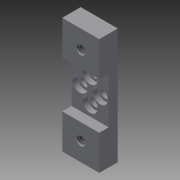
# Autodesk Inventor part: 2750-1_b
Saved by Autodesk Inventor 2014 SP2 (Build 180246200, 246)
## iProperties
Created: 2019-11-08
Part Number: 2750-1_b
Material: Generic
Catalog Web Link: www.cadenas.de
Description: 2750, 2752, 2754, 2757, 2750-Black, 2752-Black, 2754-Black, 2757-Black_b-Roller Wheel Brackets
Vendor: 8020
Document SubType Name: Modeling
Designer: psadmin
Manufacturer: 8020
Mass: 18.3475 g
Surface Area: 73.1333 cm^2
Volume: 18.3475 cm^3
Density: 1 g/cm^3
Appearance: PSOLRGB-191-191-191
Category: PARTsolutions
Company: 8020
Title: 2750-1_b
Author: Cadenas PARTsolutions
Comments: Roller Wheel Brackets
PSOL_IDENT_0: {$CADENAS_DATA\23d-libs\8020\inch\linear_motion\2750.prj},231 {VTYP=3D},{NB=2750-1_b},{LINA=2750-1_b
PSOL_IDENT_1: },{NN=2750, 2752, 2754, 2757, 2750-Black, 2752-Black, 2754-Black, 2757-Black_b},{DATE=01.10.2019 06:
PSOL_IDENT_2: 04:24},{GEOMDATE=06.12.2017 19:34:25},{VERSION=},{LINEID=10},{WBVAR=FINISH,MS},{WBNUMERIC=}  {NB=275
PSOL_IDENT_3: 0-1_b},{LINA=2750-1_b},{KT=DUMMY},{PN=2750},{MAT=Aluminum},{FINISH=CA},{MS=1},{A=3.125},{B=2.125},{C=
PSOL_IDENT_4: 1.251},{D=1.897},{E=1.5625},{F=0.669},{G=0.937},{H=0.500},{J=0.255},{K=0.500},{L=1.000},{M=0.544},{N=
PSOL_IDENT_5: 0.500},{P=0.228},{Q=1/4-20},{Q1=0.2500},{R=1/4-20},{R1=0.2570},{RCB=0.406},{RCBD=0.135},{W=.120},{FT=
PSOL_IDENT_6: 0.087},{CLR=.75,.75,.75}
NN: 2750, 2752, 2754, 2757, 2750-Black, 2752-Black, 2754-Black, 2757-Black_b
NT: Roller Wheel Brackets
NB: 2750-1_b
NBSYN: $PN.-$MS._b
LINA: 2750-1_b
PN: 2750
MAT: Aluminum
FINISH: Clear Anodize
MS: Mounting Style 1
A: 3.125
B: 2.125
C: 1.251
D: 1.897
E: 1.5625
F: 0.669
G: 0.937
H: 0.5
J: 0.255
K: 0.5
L: 1
M: 0.544
N: 0.5
P: 0.228
Q: 1/4-20
R: 1/4-20
W: .120
FT: 0.087
SUPPLIER: 8020
ARTICLENO: 2750-1_b
BOMINFO: 2750-1_b
CREATOR: CADENAS GmbH
Autodesk Inventor part; units mm, degrees
ref_plane "YZ Plane" through (0, 0, 0) normal (1, 0, 0) x (0, 1, 0)
ref_plane "XZ Plane" through (0, 0, 0) normal (0, 1, 0) x (-1, 0, 0)
ref_plane "XY Plane" through (0, 0, 0) normal (0, 0, 1) x (1, 0, 0)
sketch "Sketch_1" plane through (0, 0, 0) normal (1, 0, 0) x (0, 1, 0)
  line L0 (-15.8877, 6.477) -> (-39.6875, 6.477)
  line L1 (-39.6875, 6.477) -> (-39.6875, -6.223)
  line L2 (-39.6875, -6.223) -> (39.6875, -6.223)
  line L3 (39.6875, -6.223) -> (39.6875, 6.477)
  line L4 (39.6875, 6.477) -> (15.8877, 6.477)
  line L5 (15.8877, 6.477) -> (15.8877, 0)
  line L6 (15.8877, 0) -> (-15.8877, 0)
  line L7 (-15.8877, 0) -> (-15.8877, 6.477)
  constraints: 16 end point
extrude "Extrusion1" add sketch "Sketch_1" along normal mid plane 25.4
sketch "Sketch_2" plane through (0, 0, 0) normal (1, 0, 0) x (0, 1, 0)
  line L0 (26.9875, -6.223) -> (26.9875, 6.477)
  line L1 (26.9875, 6.477) -> (30.1625, 6.477)
  line L2 (30.1625, 6.477) -> (29.4754, 5.7899)
  line L3 (29.4754, 5.7899) -> (29.4754, -5.5359)
  line L4 (29.4754, -5.5359) -> (30.1625, -6.223)
  line L5 (30.1625, -6.223) -> (26.9875, -6.223)
  line L6 (26.9875, -6.223) -> (26.9875, 6.477)
  constraints: 14 end point
revolve "Revolution1" cut sketch "Sketch_2" angle 360 about axis through (0, 26.9875, -6.223) along (0, 0, -1)
thread "Thread1" size "1/4-20 UNC" class "2B" standard "ANSI Unified Screw Threads" full length
sketch "Sketch_3" plane through (0, 0, 0) normal (1, 0, 0) x (0, 1, 0)
  line L0 (-26.9875, -6.223) -> (-26.9875, 6.477)
  line L1 (-26.9875, 6.477) -> (-23.8125, 6.477)
  line L2 (-23.8125, 6.477) -> (-24.4996, 5.7899)
  line L3 (-24.4996, 5.7899) -> (-24.4996, -5.5359)
  line L4 (-24.4996, -5.5359) -> (-23.8125, -6.223)
  line L5 (-23.8125, -6.223) -> (-26.9875, -6.223)
  line L6 (-26.9875, -6.223) -> (-26.9875, 6.477)
  constraints: 14 end point
revolve "Revolution2" cut sketch "Sketch_3" angle 360 about axis through (0, -26.9875, -6.223) along (0, 0, -1)
thread "Thread2" size "1/4-20 UNC" class "2B" standard "ANSI Unified Screw Threads" full length
sketch "Sketch4" plane through (-12.7, -15.8877, 0) normal (0, 0, 1) x (1, 0, 0)
  point P0 (5.7912, 15.8877)
hole "Hole1" at (-6.9088, 0, 0) direction (0, 0, -1) diameter 6.5278 depth 6.223 counterbore diameter 10.3124 counterbore depth 3.429
pattern_linear "Rectangular Pattern1" count 2 spacing 10.9507 along (0.6308982, 0.7758656, 0) count 2 spacing 10.9507 along (0.6308982, -0.7758656, 0) of "Hole1"
ref_plane "screw1_XY" through (-6.9088, 0, -3.429) normal (0, 0, 1) x (1, 0, 0)
ref_plane "screw1_YZ" through (-6.9088, 0, -3.429) normal (1, 0, 0) x (0, 1, 0)
ref_plane "screw1_ZX" through (-6.9088, 0, -3.429) normal (0, 1, 0) x (0, 0, 1)
ref_plane "screw1_1_XY" through (0, 8.4963, -3.429) normal (0, 0, 1) x (1, 0, 0)
ref_plane "screw1_1_YZ" through (0, 8.4963, -3.429) normal (1, 0, 0) x (0, 1, 0)
ref_plane "screw1_1_ZX" through (0, 8.4963, -3.429) normal (0, 1, 0) x (0, 0, 1)
ref_plane "screw2_XY" through (6.9088, 0, -3.429) normal (0, 0, 1) x (1, 0, 0)
ref_plane "screw2_YZ" through (6.9088, 0, -3.429) normal (1, 0, 0) x (0, 1, 0)
ref_plane "screw2_ZX" through (6.9088, 0, -3.429) normal (0, 1, 0) x (0, 0, 1)
ref_plane "screw2_1_XY" through (0, -8.4963, -3.429) normal (0, 0, 1) x (1, 0, 0)
ref_plane "screw2_1_YZ" through (0, -8.4963, -3.429) normal (1, 0, 0) x (0, 1, 0)
ref_plane "screw2_1_ZX" through (0, -8.4963, -3.429) normal (0, 1, 0) x (0, 0, 1)
ref_plane "to_dummy_XY" through (0, 0, -6.223) normal (0, 0, 1) x (1, 0, 0)
ref_plane "to_dummy_YZ" through (0, 0, -6.223) normal (1, 0, 0) x (0, 1, 0)
ref_plane "to_dummy_ZX" through (0, 0, -6.223) normal (0, 1, 0) x (0, 0, 1)
ref_plane "to_screw1_XY" through (0, 26.9875, 6.477) normal (0, 0, 1) x (1, 0, 0)
ref_plane "to_screw1_YZ" through (0, 26.9875, 6.477) normal (1, 0, 0) x (0, 1, 0)
ref_plane "to_screw1_ZX" through (0, 26.9875, 6.477) normal (0, 1, 0) x (0, 0, 1)
ref_plane "to_screw2_XY" through (0, -26.9875, 6.477) normal (0, 0, 1) x (1, 0, 0)
ref_plane "to_screw2_YZ" through (0, -26.9875, 6.477) normal (1, 0, 0) x (0, 1, 0)
ref_plane "to_screw2_ZX" through (0, -26.9875, 6.477) normal (0, 1, 0) x (0, 0, 1)
body "Solid1"
